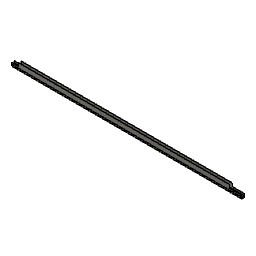
Correção Janela traseiro saveiro v1 (Autodesk Fusion 360 design; units mm, degrees)
Autodesk Fusion 360 part; units mm, degrees
sketch "Esboço1" plane through (0, 0, 0) normal (0, 1, 0) x (1, 0, 0)
  line L0 (0, 0) -> (363, 0)
  line L1 (363, 0) -> (363, -5)
  line L2 (363, -5) -> (344, -5)
  line L3 (344, -5) -> (344, -10)
  line L4 (344, -10) -> (11, -10)
  line L5 (11, -10) -> (11, -5)
  line L6 (11, -5) -> (0, -5)
  line L7 (0, -5) -> (0, 0)
  dimension "d1" = 363
  dimension "d2" = 5
  dimension "d3" = 19
  dimension "d6" = 333
  dimension "d7" = 11
  dimension "d8" = 10
  constraint coincident L0.start L7.end
  constraint horizontal L0
  constraint perpendicular L0 L1
  constraint perpendicular L1 L2
  constraint perpendicular L2 L3
  constraint perpendicular L3 L4
  constraint perpendicular L4 L5
  constraint perpendicular L5 L6
  constraint perpendicular L0 L7
  measures "d1" distance of L0.start L0.end
  measures "d2" distance of L0.end L1.end
  measures "d3" distance of L1.end L2.end
  measures "d6" distance of L3.end L4.end
  measures "d7" distance of L5.end L6.end
  measures "d8" vertical distance of L0.end L3.end
extrude "Extrusão1" add sketch "Esboço1" along normal blind 4.4
ref_plane "Plano de trabalho1" through (0, 2.2, 0) normal (0, 1, 0) x (0, 0, 1)
sketch "Esboço2" plane through (0, 2.2, 0) normal (0, 1, 0) x (1, 0, 0)
  line L0 (0, -10.1764) -> (363, -10.1764)
  line L1 (363, -10.1764) -> (363, -2.1764)
  line L2 (363, -2.1764) -> (0, -2.1764)
  line L3 (0, -2.1764) -> (0, -10.1764)
  dimension "d12" = 8
  dimension "d13" = 363
  constraint horizontal L0
  constraint vertical L1
  constraint horizontal L2
  constraint vertical L3
  measures "d12" distance of L0.start L2.end
  measures "d13" distance of L0.start L0.end
extrude "Extrusão2" cut sketch "Esboço2" along normal mid plane 4
